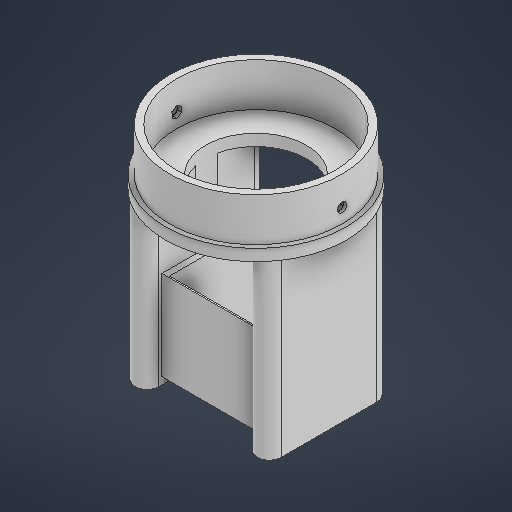
# Autodesk Inventor part: cam_mount90
Saved by Autodesk Inventor 2027 (Build 310192060, 192F)
## iProperties
Created: 2026-07-16
Part Number: cam_mount90
Material: Generic
Document SubType Name: Modeling
Designer: farde
Density: 1 g/cm^3
Appearance: Default
Author: farde
Autodesk Inventor part; units mm, degrees
ref_plane "YZ Plane" through (0, 0, 0) normal (1, 0, 0) x (0, 1, 0)
ref_plane "XZ Plane" through (0, 0, 0) normal (0, 1, 0) x (-1, 0, 0)
ref_plane "XY Plane" through (0, 0, 0) normal (0, 0, 1) x (1, 0, 0)
sketch "Sketch1" plane through (0, 0, 0) normal (0, 1, 0) x (-1, 0, 0)
  circle A0 centre (0, 0) radius 29.85
  circle A1 centre (0, 0) radius 27.5
  dimension "d0" = 59.7
  dimension "d1" = 55
  constraints: 2 centre point, 2 coincident
  measures "d0" diameter of A0
  measures "d1" diameter of A1
extrude "Extrusion1" add sketch "Sketch1" along normal blind 15
sketch "Sketch2" plane through (0, 0, 0) normal (0, 1, 0) x (-1, 0, 0)
  circle A0 centre (0, 0) radius 31.4135
  circle A1 centre (0, 0) radius 28.9404
  circle A2 centre (0, 0) radius 31.4135
  circle A3 centre (0, 0) radius 20.0919
  dimension "d6" = 40.1837
  constraints: 4 centre point, 4 coincident, 1 concentric
  measures "d6" diameter of A3
extrude "Extrusion2" add sketch "Sketch2" against normal blind 4 contours A0 | A1 | A3
sketch "Sketch3" plane through (0, -4, 0) normal (0, -1, 0) x (1, 0, 0)
  line L0 (21.2066, 16.5968) -> (21.2066, -16.5968) construction
  line L1 (17.0959, 16.5968) -> (17.0959, -16.5968)
  line L2 (25.3174, -16.5968) -> (25.3174, 16.5968)
  arc A0 (25.3174, 16.5968) -> (17.0959, 16.5968) centre (21.2066, 16.5968) ccw
  arc A1 (17.0959, -16.5968) -> (25.3174, -16.5968) centre (21.2066, -16.5968) ccw
  point P0 (0, 0)
  point P1 (21.2066, 0)
  dimension "d28" = 8.2215
  constraints: 8 end point, 4 point on circle, 4 tangent, 2 centre point, 1 midpoint, 1 parallel, 1 vertical
  measures "d28" distance between parallel lines of L1 L2
extrude "Extrusion3" add sketch "Sketch3" along normal blind 60
mirror "Mirror1" about plane through (0, 0, 0) normal (1, 0, 0) of "Extrusion3"
sketch "Sketch4" plane through (0, 0, 0) normal (0, 1, 0) x (1, 0, 0)
  circle A0 centre (0, 0) radius 17.5
  dimension "d11" = 35
  constraints: 1 centre point, 1 coincident
  measures "d11" diameter of A0
extrude "Extrusion4" cut sketch "Sketch4" against normal blind 60
sketch "Sketch5" plane through (17.0959, -64, -16.5968) normal (-1, 0, 0) x (0, 0, 1)
  line L0 (32.0968, 2.4749) -> (1.0968, 2.4749)
  line L1 (1.0968, 2.4749) -> (1.0968, 33.4749)
  line L2 (1.0968, 33.4749) -> (32.0968, 33.4749)
  line L3 (32.0968, 33.4749) -> (32.0968, 2.4749)
  line L4 (32.0968, 2.4749) -> (1.0968, 33.4749) construction
  line L5 (1.0968, 2.4749) -> (32.0968, 33.4749) construction
  point P0 (16.5968, 64)
  point P1 (16.5968, 17.9749)
  dimension "d12" = 31
  dimension "d13" = 31
  constraints: 12 end point, 2 midpoint, 2 parallel, 1 horizontal, 1 perpendicular
  measures "d12" distance of L1.end L2.end
  measures "d13" distance of L0.end L1.end
extrude "Extrusion5" add sketch "Sketch5" along normal blind 36.1875
sketch "Sketch6" plane through (17.0959, -61.5251, -15.5) normal (0, -1, 0) x (1, 0, 0)
  point P0 (-17.0959, 15.5)
sketch "Sketch7" plane through (17.0959, -61.5251, -15.5) normal (0, -1, 0) x (1, 0, 0)
  line L0 (-32.0959, 30.5) -> (-2.0959, 30.5)
  line L1 (-2.0959, 30.5) -> (-2.0959, 0.5)
  line L2 (-2.0959, 0.5) -> (-32.0959, 0.5)
  line L3 (-32.0959, 0.5) -> (-32.0959, 30.5)
  line L4 (-32.0959, 30.5) -> (-2.0959, 0.5) construction
  line L5 (-2.0959, 30.5) -> (-32.0959, 0.5) construction
  point P0 (-17.0959, 15.5)
  dimension "d16" = 30
  dimension "d17" = 30
  constraints: 12 end point, 2 midpoint, 2 parallel, 1 horizontal, 1 perpendicular
  measures "d16" distance of L1.end L2.end
  measures "d17" distance of L0.end L1.end
extrude "Extrusion6" cut sketch "Sketch7" against normal blind 33.0125
sketch "Sketch8" plane through (-25.3174, -64, -16.5968) normal (-1, 0, 0) x (0, 0, 1)
  line L0 (27.33, 20.5912) -> (-74.1146, 20.5912) construction
  line L1 (-74.1146, 20.5912) -> (-74.1146, 156.4096) construction
  line L2 (-74.1146, 156.4096) -> (27.33, 156.4096) construction
  line L3 (27.33, 156.4096) -> (27.33, 20.5912) construction
  spline S0 degree 2 poles (26.738, 25.0947) (26.738, 24.0904) (26.0826, 22.4201) (25.5117, 21.8175) knots 0 0 0 1 2 2 2
  spline S1 degree 2 poles (25.5117, 21.8175) (24.9726, 21.2361) (23.3974, 20.5912) (22.5939, 20.5912) knots 0 0 0 1 2 2 2
  spline S2 degree 2 poles (22.5939, 20.5912) (21.6953, 20.5912) (20.2364, 21.1938) (19.6973, 21.7647) knots 0 0 0 1 2 2 2
  spline S3 degree 2 poles (19.6973, 21.7647) (19.0207, 22.4835) (18.2807, 24.8093) (18.2807, 26.5959) knots 0 0 0 1 2 2 2
  spline S4 degree 2 poles (18.2807, 26.5959) (18.2807, 28.2134) (19.0101, 31.11) (19.7184, 32.072) knots 0 0 0 1 2 2 2
  spline S5 degree 2 poles (19.7184, 32.072) (20.469, 33.0869) (22.5834, 34.1547) (24.1268, 34.1547) knots 0 0 0 1 2 2 2
  spline S6 degree 2 poles (24.1268, 34.1547) (24.4757, 34.1547) (25.2686, 34.0807) (25.6069, 33.9749) knots 0 0 0 1 2 2 2
  line L4 (25.6069, 33.9749) -> (25.6069, 32.294)
  line L5 (25.6069, 32.294) -> (25.5223, 32.294)
  spline S7 degree 2 poles (25.5223, 32.294) (25.3003, 32.4209) (24.37, 32.6429) (23.8942, 32.6429) knots 0 0 0 1 2 2 2
  spline S8 degree 2 poles (23.8942, 32.6429) (22.1816, 32.6429) (20.2259, 30.3806) (20.0884, 28.2874) knots 0 0 0 1 2 2 2
  spline S9 degree 2 poles (20.0884, 28.2874) (20.7862, 28.7631) (22.0548, 29.1965) (22.8054, 29.1965) knots 0 0 0 1 2 2 2
  spline S10 degree 2 poles (22.8054, 29.1965) (23.5242, 29.1965) (24.7188, 28.8794) (25.3214, 28.4248) knots 0 0 0 1 2 2 2
  spline S11 degree 2 poles (25.3214, 28.4248) (26.0191, 27.8857) (26.738, 26.247) (26.738, 25.0947) knots 0 0 0 1 2 2 2
  spline S12 degree 2 poles (20.0462, 26.2048) (20.0462, 24.8833) (20.5325, 23.213) (20.9659, 22.7584) knots 0 0 0 1 2 2 2
  spline S13 degree 2 poles (20.9659, 22.7584) (21.3465, 22.3355) (22.1393, 22.0184) (22.6045, 22.0184) knots 0 0 0 1 2 2 2
  spline S14 degree 2 poles (22.6045, 22.0184) (23.6828, 22.0184) (24.962, 23.5618) (24.962, 25.0207) knots 0 0 0 1 2 2 2
  spline S15 degree 2 poles (24.962, 25.0207) (24.962, 25.8453) (24.5391, 26.9131) (24.074, 27.2936) knots 0 0 0 1 2 2 2
  spline S16 degree 2 poles (24.074, 27.2936) (23.7357, 27.5685) (22.9005, 27.7482) (22.4142, 27.7482) knots 0 0 0 1 2 2 2
  spline S17 degree 2 poles (22.4142, 27.7482) (21.8539, 27.7482) (20.5642, 27.3571) (20.0779, 27.0293) knots 0 0 0 1 2 2 2
  spline S18 degree 2 poles (20.0779, 27.0293) (20.0673, 26.9025) (20.0462, 26.469) (20.0462, 26.2048) knots 0 0 0 1 2 2 2
  spline S19 degree 2 poles (8.4702, 27.3782) (8.4702, 30.888) (10.5105, 34.1758) (12.6354, 34.1758) knots 0 0 0 1 2 2 2
  spline S20 degree 2 poles (12.6354, 34.1758) (14.792, 34.1758) (16.8112, 30.8246) (16.8112, 27.3888) knots 0 0 0 1 2 2 2
  spline S21 degree 2 poles (16.8112, 27.3888) (16.8112, 23.8578) (14.7709, 20.5912) (12.6354, 20.5912) knots 0 0 0 1 2 2 2
  spline S22 degree 2 poles (12.6354, 20.5912) (10.4894, 20.5912) (8.4702, 23.9741) (8.4702, 27.3782) knots 0 0 0 1 2 2 2
  spline S23 degree 2 poles (10.7114, 31.3532) (10.4576, 30.7083) (10.2462, 28.7208) (10.2462, 27.3782) knots 0 0 0 1 2 2 2
  spline S24 degree 2 poles (10.2462, 27.3782) (10.2462, 26.0356) (10.4576, 24.0587) (10.7219, 23.3927) knots 0 0 0 1 2 2 2
  spline S25 degree 2 poles (10.7219, 23.3927) (10.9862, 22.7267) (11.906, 22.0395) (12.6354, 22.0395) knots 0 0 0 1 2 2 2
  spline S26 degree 2 poles (12.6354, 22.0395) (13.3649, 22.0395) (14.3057, 22.7267) (14.5806, 23.4138) knots 0 0 0 1 2 2 2
  spline S27 degree 2 poles (14.5806, 23.4138) (14.8449, 24.0799) (15.0352, 26.1096) (15.0352, 27.3888) knots 0 0 0 1 2 2 2
  spline S28 degree 2 poles (15.0352, 27.3888) (15.0352, 28.7631) (14.866, 30.6026) (14.5912, 31.3214) knots 0 0 0 1 2 2 2
  spline S29 degree 2 poles (14.5912, 31.3214) (14.3375, 31.998) (13.3966, 32.7275) (12.6354, 32.7275) knots 0 0 0 1 2 2 2
  spline S30 degree 2 poles (12.6354, 32.7275) (11.9165, 32.7275) (10.9757, 32.0403) (10.7114, 31.3532) knots 0 0 0 1 2 2 2
  spline S31 degree 2 poles (0.1926, 23.9636) (0.1926, 25.3696) (2.1166, 27.2936) (3.5226, 27.2936) knots 0 0 0 1 2 2 2
  spline S32 degree 2 poles (3.5226, 27.2936) (4.9181, 27.2936) (6.8633, 25.3802) (6.8633, 23.9636) knots 0 0 0 1 2 2 2
  spline S33 degree 2 poles (6.8633, 23.9636) (6.8633, 22.5575) (4.9392, 20.6335) (3.5226, 20.6335) knots 0 0 0 1 2 2 2
  spline S34 degree 2 poles (3.5226, 20.6335) (2.1166, 20.6335) (0.1926, 22.5575) (0.1926, 23.9636) knots 0 0 0 1 2 2 2
  spline S35 degree 2 poles (1.5669, 23.9636) (1.5669, 23.1178) (2.6875, 21.9655) (3.5226, 21.9655) knots 0 0 0 1 2 2 2
  spline S36 degree 2 poles (3.5226, 21.9655) (4.3684, 21.9655) (5.489, 23.1178) (5.489, 23.9636) knots 0 0 0 1 2 2 2
  spline S37 degree 2 poles (5.489, 23.9636) (5.489, 24.8199) (4.3472, 25.9616) (3.5226, 25.9616) knots 0 0 0 1 2 2 2
  spline S38 degree 2 poles (3.5226, 25.9616) (2.6875, 25.9616) (1.5669, 24.7987) (1.5669, 23.9636) knots 0 0 0 1 2 2 2
  point P0 (16.5968, 64)
  constraints: 2 other
sketch "Sketch9" plane through (0, 0, 0) normal (1, 0, 0) x (0, 1, 0)
  circle A0 centre (5, 0) radius 1.6
  line L0 (0, -31.4135) -> (0, 31.4135) projected
  point P0 (0, 0)
  dimension "d22" = 3.2
  dimension "d25" = 5
  constraints: 1 centre point
  measures "d22" diameter of A0
  measures "d25" distance from line of L0 A0.centre
extrude "Extrusion8" cut sketch "Sketch9" along normal mid plane 78.2
sketch "Sketch10" plane through (0, 0, 0) normal (1, 0, 0) x (0, 1, 0)
  line L0 (5.9683, -1.6274) -> (4.0574, -1.6823)
  line L1 (4.0574, -1.6823) -> (3.0544, -0.0549)
  line L2 (3.0544, -0.0549) -> (3.9623, 1.6274)
  line L3 (3.9623, 1.6274) -> (5.8731, 1.6823)
  line L4 (5.8731, 1.6823) -> (6.8761, 0.0549)
  line L5 (6.8761, 0.0549) -> (5.9683, -1.6274)
  point P0 (0, 0)
  point P1 (4.9653, 0)
  constraints: 12 end point, 13 other
extrude "Extrusion9" cut sketch "Sketch10" along normal mid plane 57.5625
sketch "Sketch11" plane through (-25.3174, -64, -16.5968) normal (-1, 0, 0) x (0, 0, 1)
  line L0 (23.7481, 35.1884) -> (-5.73, 35.1884) construction
  line L1 (-5.73, 35.1884) -> (-5.73, 39.6022) construction
  line L2 (-5.73, 39.6022) -> (23.7481, 39.6022) construction
  line L3 (23.7481, 39.6022) -> (23.7481, 35.1884) construction
  line L4 (21.6116, 35.7812) -> (22.9306, 38.3722)
  line L5 (22.9306, 38.3722) -> (23.3653, 38.3722)
  line L6 (23.3653, 38.3722) -> (21.9722, 35.6824)
  line L7 (21.9722, 35.6824) -> (23.5456, 35.6824)
  line L8 (23.5456, 35.6824) -> (23.5456, 35.3242)
  line L9 (23.5456, 35.3242) -> (21.6116, 35.3242)
  line L10 (21.6116, 35.3242) -> (21.6116, 35.7812)
  line L11 (19.9715, 35.1884) -> (21.1645, 39.0342)
  line L12 (21.1645, 39.0342) -> (21.5103, 39.0342)
  line L13 (21.5103, 39.0342) -> (20.3222, 35.1884)
  line L14 (20.3222, 35.1884) -> (19.9715, 35.1884)
  line L15 (17.7559, 38.3722) -> (19.6356, 38.3722)
  line L16 (19.6356, 38.3722) -> (19.6356, 37.94)
  spline S0 degree 2 poles (19.6356, 37.94) (19.433, 37.7498) (19.0724, 37.3966) (18.8995, 37.2064) knots 0 0 0 1 2 2 2
  spline S1 degree 2 poles (18.8995, 37.2064) (18.5512, 36.8235) (18.2968, 36.3641) (18.2968, 36.1196) knots 0 0 0 1 2 2 2
  spline S2 degree 2 poles (18.2968, 36.1196) (18.2968, 35.9911) (18.3759, 35.7985) (18.4475, 35.7367) knots 0 0 0 1 2 2 2
  spline S3 degree 2 poles (18.4475, 35.7367) (18.5191, 35.675) (18.7068, 35.6132) (18.8205, 35.6132) knots 0 0 0 1 2 2 2
  spline S4 degree 2 poles (18.8205, 35.6132) (18.9291, 35.6132) (19.1514, 35.6676) (19.2527, 35.7096) knots 0 0 0 1 2 2 2
  spline S5 degree 2 poles (19.2527, 35.7096) (19.3392, 35.7441) (19.4997, 35.8429) (19.5491, 35.8775) knots 0 0 0 1 2 2 2
  line L17 (19.5491, 35.8775) -> (19.5713, 35.8775)
  line L18 (19.5713, 35.8775) -> (19.5713, 35.4428)
  spline S6 degree 2 poles (19.5713, 35.4428) (19.4454, 35.381) (18.9934, 35.26) (18.7908, 35.26) knots 0 0 0 1 2 2 2
  spline S7 degree 2 poles (18.7908, 35.26) (18.3635, 35.26) (17.8819, 35.712) (17.8819, 36.0973) knots 0 0 0 1 2 2 2
  spline S8 degree 2 poles (17.8819, 36.0973) (17.8819, 36.2777) (17.9658, 36.579) (18.0399, 36.7074) knots 0 0 0 1 2 2 2
  spline S9 degree 2 poles (18.0399, 36.7074) (18.114, 36.8408) (18.3289, 37.1026) (18.4475, 37.2286) knots 0 0 0 1 2 2 2
  spline S10 degree 2 poles (18.4475, 37.2286) (18.6401, 37.4386) (19.1119, 37.8881) (19.2527, 38.019) knots 0 0 0 1 2 2 2
  line L19 (19.2527, 38.019) -> (17.7559, 38.019)
  line L20 (17.7559, 38.019) -> (17.7559, 38.3722)
  spline S11 degree 2 poles (15.4514, 36.8482) (15.4514, 37.6683) (15.9281, 38.4365) (16.4245, 38.4365) knots 0 0 0 1 2 2 2
  spline S12 degree 2 poles (16.4245, 38.4365) (16.9284, 38.4365) (17.4002, 37.6535) (17.4002, 36.8507) knots 0 0 0 1 2 2 2
  spline S13 degree 2 poles (17.4002, 36.8507) (17.4002, 36.0257) (16.9235, 35.2625) (16.4245, 35.2625) knots 0 0 0 1 2 2 2
  spline S14 degree 2 poles (16.4245, 35.2625) (15.9231, 35.2625) (15.4514, 36.0529) (15.4514, 36.8482) knots 0 0 0 1 2 2 2
  spline S15 degree 2 poles (15.975, 37.777) (15.9157, 37.6263) (15.8663, 37.1619) (15.8663, 36.8482) knots 0 0 0 1 2 2 2
  spline S16 degree 2 poles (15.8663, 36.8482) (15.8663, 36.5345) (15.9157, 36.0726) (15.9775, 35.917) knots 0 0 0 1 2 2 2
  spline S17 degree 2 poles (15.9775, 35.917) (16.0392, 35.7614) (16.2541, 35.6009) (16.4245, 35.6009) knots 0 0 0 1 2 2 2
  spline S18 degree 2 poles (16.4245, 35.6009) (16.595, 35.6009) (16.8148, 35.7614) (16.879, 35.922) knots 0 0 0 1 2 2 2
  spline S19 degree 2 poles (16.879, 35.922) (16.9408, 36.0776) (16.9852, 36.5518) (16.9852, 36.8507) knots 0 0 0 1 2 2 2
  spline S20 degree 2 poles (16.9852, 36.8507) (16.9852, 37.1718) (16.9457, 37.6016) (16.8815, 37.7695) knots 0 0 0 1 2 2 2
  spline S21 degree 2 poles (16.8815, 37.7695) (16.8222, 37.9276) (16.6024, 38.0981) (16.4245, 38.0981) knots 0 0 0 1 2 2 2
  spline S22 degree 2 poles (16.4245, 38.0981) (16.2566, 38.0981) (16.0367, 37.9375) (15.975, 37.777) knots 0 0 0 1 2 2 2
  line L21 (13.794, 35.1884) -> (14.987, 39.0342)
  line L22 (14.987, 39.0342) -> (15.3328, 39.0342)
  line L23 (15.3328, 39.0342) -> (14.1447, 35.1884)
  line L24 (14.1447, 35.1884) -> (13.794, 35.1884)
  line L25 (11.5784, 38.3722) -> (13.4581, 38.3722)
  line L26 (13.4581, 38.3722) -> (13.4581, 37.94)
  spline S23 degree 2 poles (13.4581, 37.94) (13.2555, 37.7498) (12.8949, 37.3966) (12.722, 37.2064) knots 0 0 0 1 2 2 2
  spline S24 degree 2 poles (12.722, 37.2064) (12.3737, 36.8235) (12.1193, 36.3641) (12.1193, 36.1196) knots 0 0 0 1 2 2 2
  spline S25 degree 2 poles (12.1193, 36.1196) (12.1193, 35.9911) (12.1983, 35.7985) (12.27, 35.7367) knots 0 0 0 1 2 2 2
  spline S26 degree 2 poles (12.27, 35.7367) (12.3416, 35.675) (12.5293, 35.6132) (12.6429, 35.6132) knots 0 0 0 1 2 2 2
  spline S27 degree 2 poles (12.6429, 35.6132) (12.7516, 35.6132) (12.9739, 35.6676) (13.0752, 35.7096) knots 0 0 0 1 2 2 2
  spline S28 degree 2 poles (13.0752, 35.7096) (13.1616, 35.7441) (13.3222, 35.8429) (13.3716, 35.8775) knots 0 0 0 1 2 2 2
  line L27 (13.3716, 35.8775) -> (13.3938, 35.8775)
  line L28 (13.3938, 35.8775) -> (13.3938, 35.4428)
  spline S29 degree 2 poles (13.3938, 35.4428) (13.2679, 35.381) (12.8158, 35.26) (12.6133, 35.26) knots 0 0 0 1 2 2 2
  spline S30 degree 2 poles (12.6133, 35.26) (12.186, 35.26) (11.7043, 35.712) (11.7043, 36.0973) knots 0 0 0 1 2 2 2
  spline S31 degree 2 poles (11.7043, 36.0973) (11.7043, 36.2777) (11.7883, 36.579) (11.8624, 36.7074) knots 0 0 0 1 2 2 2
  spline S32 degree 2 poles (11.8624, 36.7074) (11.9365, 36.8408) (12.1514, 37.1026) (12.27, 37.2286) knots 0 0 0 1 2 2 2
  spline S33 degree 2 poles (12.27, 37.2286) (12.4626, 37.4386) (12.9344, 37.8881) (13.0752, 38.019) knots 0 0 0 1 2 2 2
  line L29 (13.0752, 38.019) -> (11.5784, 38.019)
  line L30 (11.5784, 38.019) -> (11.5784, 38.3722)
  spline S34 degree 2 poles (9.2442, 37.3842) (9.2442, 37.6189) (9.3998, 38.0165) (9.5307, 38.1499) knots 0 0 0 1 2 2 2
  spline S35 degree 2 poles (9.5307, 38.1499) (9.6666, 38.2907) (10.0074, 38.4365) (10.2125, 38.4365) knots 0 0 0 1 2 2 2
  spline S36 degree 2 poles (10.2125, 38.4365) (10.4175, 38.4365) (10.7559, 38.2981) (10.8843, 38.1598) knots 0 0 0 1 2 2 2
  spline S37 degree 2 poles (10.8843, 38.1598) (11.0424, 37.9943) (11.2202, 37.4386) (11.2202, 37.0335) knots 0 0 0 1 2 2 2
  spline S38 degree 2 poles (11.2202, 37.0335) (11.2202, 36.6358) (11.0572, 35.9961) (10.8868, 35.759) knots 0 0 0 1 2 2 2
  spline S39 degree 2 poles (10.8868, 35.759) (10.7213, 35.5268) (10.1976, 35.2674) (9.8543, 35.2674) knots 0 0 0 1 2 2 2
  spline S40 degree 2 poles (9.8543, 35.2674) (9.753, 35.2674) (9.5752, 35.2872) (9.5085, 35.3094) knots 0 0 0 1 2 2 2
  line L31 (9.5085, 35.3094) -> (9.5085, 35.7021)
  line L32 (9.5085, 35.7021) -> (9.5258, 35.7021)
  spline S41 degree 2 poles (9.5258, 35.7021) (9.5826, 35.6725) (9.7901, 35.6206) (9.9086, 35.6206) knots 0 0 0 1 2 2 2
  spline S42 degree 2 poles (9.9086, 35.6206) (10.289, 35.6206) (10.7559, 36.1344) (10.8003, 36.6383) knots 0 0 0 1 2 2 2
  spline S43 degree 2 poles (10.8003, 36.6383) (10.6546, 36.537) (10.3483, 36.4259) (10.1655, 36.4259) knots 0 0 0 1 2 2 2
  spline S44 degree 2 poles (10.1655, 36.4259) (9.9877, 36.4259) (9.7209, 36.4975) (9.5752, 36.6062) knots 0 0 0 1 2 2 2
  spline S45 degree 2 poles (9.5752, 36.6062) (9.4072, 36.7321) (9.2442, 37.1224) (9.2442, 37.3842) knots 0 0 0 1 2 2 2
  spline S46 degree 2 poles (9.6592, 37.4015) (9.6592, 37.2138) (9.758, 36.9594) (9.8666, 36.8705) knots 0 0 0 1 2 2 2
  spline S47 degree 2 poles (9.8666, 36.8705) (9.9482, 36.8062) (10.1507, 36.7642) (10.2569, 36.7642) knots 0 0 0 1 2 2 2
  spline S48 degree 2 poles (10.2569, 36.7642) (10.4002, 36.7642) (10.6694, 36.8507) (10.8003, 36.9322) knots 0 0 0 1 2 2 2
  spline S49 degree 2 poles (10.8003, 36.9322) (10.8028, 36.9767) (10.8077, 37.0607) (10.8077, 37.1249) knots 0 0 0 1 2 2 2
  spline S50 degree 2 poles (10.8077, 37.1249) (10.8077, 37.441) (10.6842, 37.8288) (10.5904, 37.9301) knots 0 0 0 1 2 2 2
  spline S51 degree 2 poles (10.5904, 37.9301) (10.5039, 38.0264) (10.3162, 38.103) (10.21, 38.103) knots 0 0 0 1 2 2 2
  spline S52 degree 2 poles (10.21, 38.103) (9.963, 38.103) (9.6592, 37.7523) (9.6592, 37.4015) knots 0 0 0 1 2 2 2
  point P0 (16.5968, 64)
  constraints: 2 other
emboss "Emboss1" sketch "Sketch11" operation add depth 1 direction (1, 0, 0)
emboss "Emboss2" sketch "Sketch8" operation add depth 1 direction (1, 0, 0)
body "Solid1"
